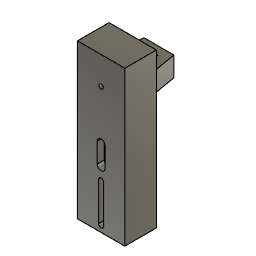
Seitenhalterung für vorne links v17 (Autodesk Fusion 360 design; units mm, degrees)
Autodesk Fusion 360 part; units mm, degrees
sketch "Skizze1" plane through (0, 0, 0) normal (0, 0, 1) x (1, 0, 0)
  line L0 (30, 20) -> (-30, 20)
  line L1 (-30, 20) -> (-30, -20)
  line L2 (-30, -20) -> (30, -20)
  line L3 (30, -20) -> (30, 20)
  line L4 (30, 20) -> (-30, -20) construction
  line L5 (-30, 20) -> (30, -20) construction
  dimension "d2" = 60
  dimension "d3" = 40
  constraint perpendicular L0 L1
  constraint parallel L0 L2
  constraint parallel L1 L3
  constraint horizontal L0
  constraint coincident L4 origin
  constraint coincident L5 origin
  measures "d2" distance of L1.end L2.end
  measures "d3" distance of L0.end L1.end
extrude "Extrusion1" add sketch "Skizze1" along normal blind 195 makes body 1
sketch "Skizze3" plane through (0, -20, 0) normal (0, -1, 0) x (1, 0, 0)
  line L0 (-30, 0) -> (30, 0)
  line L1 (30, 0) -> (30, 195)
  line L2 (30, 195) -> (-30, 195)
  line L3 (-30, 195) -> (-30, 0)
  line L4 (3.1, 8.1) -> (3.1, 56.9)
  arc A0 (3.1, 56.9) -> (-3.1, 56.9) centre (0, 56.9) ccw
  line L5 (-3.1, 56.9) -> (-3.1, 8.1)
  arc A1 (-3.1, 8.1) -> (3.1, 8.1) centre (0, 8.1) ccw
  line L6 (0, 5) -> (0, 60) construction
  line L7 (2.5, 72.5) -> (2.5, 97.5)
  arc A2 (2.5, 97.5) -> (-2.5, 97.5) centre (0, 97.5) ccw
  line L8 (-2.5, 97.5) -> (-2.5, 72.5)
  arc A3 (-2.5, 72.5) -> (2.5, 72.5) centre (0, 72.5) ccw
  line L9 (0, 70) -> (0, 100) construction
  point P0 (0, 195)
  dimension "d52" = 6.2
  dimension "d53" = 5
  constraint midpoint L2 P0
  constraint tangent L4 A0
  constraint tangent A0 L5
  constraint parallel L4 L5
  constraint tangent L5 A1
  constraint tangent L4 A1
  constraint midpoint A1 L6.start
  constraint midpoint A0 L6.end
  constraint vertical L6
  constraint tangent L7 A2
  constraint tangent A2 L8
  constraint parallel L7 L8
  constraint tangent L8 A3
  constraint tangent L7 A3
  constraint midpoint A3 L9.start
  constraint midpoint A2 L9.end
  constraint parallel L3 L9
  measures "d52" diameter of A0
  measures "d53" diameter of A2
extrude "Extrusion2" cut sketch "Skizze3" against normal blind 40 contours L4 A0 L5 A1 | L7 A2 L8 A3 bodies 1
sketch "Skizze4" plane through (30, 0, 0) normal (1, 0, 0) x (0, 1, 0)
  line L0 (-20, 0) -> (20, 0)
  line L1 (20, 0) -> (20, 195)
  line L2 (20, 195) -> (-20, 195)
  line L3 (-20, 195) -> (-20, 0)
  circle A0 centre (0, 174.5) radius 4.15
  dimension "d12" = 8.3
  measures "d12" diameter of A0
extrude "Extrusion3" add sketch "Skizze4" against normal blind 60 separate body contours A0 makes body 2
sketch "Skizze6" plane through (0, 0, 0) normal (0, 1, 0) x (1, 0, 0)
sketch "Skizze7" plane through (0, 20, 0) normal (0, 1, 0) x (-1, 0, 0)
  line L0 (-30, 0) -> (30, 0)
  line L1 (30, 0) -> (30, 195)
  line L2 (30, 195) -> (-30, 195)
  line L3 (-30, 195) -> (-30, 0)
  circle A0 centre (0, 160) radius 2.75
  line L4 (-2.5, 72.5) -> (-2.5, 97.5)
  arc A1 (2.5, 97.5) -> (-2.5, 97.5) centre (0, 97.5) ccw
  line L5 (2.5, 97.5) -> (2.5, 72.5)
  arc A2 (-2.5, 72.5) -> (2.5, 72.5) centre (0, 72.5) ccw
  line L6 (-3.1, 8.1) -> (-3.1, 56.9)
  arc A3 (3.1, 56.9) -> (-3.1, 56.9) centre (0, 56.9) ccw
  line L7 (3.1, 56.9) -> (3.1, 8.1)
  arc A4 (-3.1, 8.1) -> (3.1, 8.1) centre (0, 8.1) ccw
  dimension "d17" = 5.5
  measures "d17" diameter of A0
extrude "Extrusion4" cut sketch "Skizze7" against normal blind 40 contours A0 bodies 1
sketch "Skizze8" plane through (0, 20, 0) normal (0, 1, 0) x (-1, 0, 0)
  circle A0 centre (0, 160) radius 2.75
  line L0 (-30, 0) -> (30, 0)
  line L1 (30, 0) -> (30, 195)
  line L2 (30, 195) -> (-30, 195)
  line L3 (-30, 195) -> (-30, 0)
  circle A1 centre (0, 160) radius 6.65
  line L4 (-2.5, 72.5) -> (-2.5, 97.5)
  arc A2 (2.5, 97.5) -> (-2.5, 97.5) centre (0, 97.5) ccw
  line L5 (2.5, 97.5) -> (2.5, 72.5)
  arc A3 (-2.5, 72.5) -> (2.5, 72.5) centre (0, 72.5) ccw
  line L6 (-3.1, 8.1) -> (-3.1, 56.9)
  arc A4 (3.1, 56.9) -> (-3.1, 56.9) centre (0, 56.9) ccw
  line L7 (3.1, 56.9) -> (3.1, 8.1)
  arc A5 (-3.1, 8.1) -> (3.1, 8.1) centre (0, 8.1) ccw
  dimension "d20" = 13.3
  constraint concentric A0 A1
  measures "d20" diameter of A1
extrude "Extrusion5" cut sketch "Skizze8" against normal blind 4 contours A1 bodies 1
sketch "Skizze10" plane through (0, 20, 0) normal (0, 1, 0) x (-1, 0, 0)
  circle A0 centre (0, 160) radius 6.65
  line L0 (-30, 0) -> (30, 0)
  line L1 (30, 0) -> (30, 195)
  line L2 (30, 195) -> (-30, 195)
  line L3 (-30, 195) -> (-30, 0)
  line L4 (-14, 172.5) -> (-21, 172.5)
  line L5 (-21, 172.5) -> (-21, 147.5)
  line L6 (-21, 147.5) -> (-14, 147.5)
  line L7 (-14, 147.5) -> (-14, 172.5)
  line L8 (-2.5, 72.5) -> (-2.5, 97.5)
  arc A1 (2.5, 97.5) -> (-2.5, 97.5) centre (0, 97.5) ccw
  line L9 (2.5, 97.5) -> (2.5, 72.5)
  arc A2 (-2.5, 72.5) -> (2.5, 72.5) centre (0, 72.5) ccw
  line L10 (-3.1, 8.1) -> (-3.1, 56.9)
  arc A3 (3.1, 56.9) -> (-3.1, 56.9) centre (0, 56.9) ccw
  line L11 (3.1, 56.9) -> (3.1, 8.1)
  arc A4 (-3.1, 8.1) -> (3.1, 8.1) centre (0, 8.1) ccw
  dimension "d27" = 7
  dimension "d28" = 25
  constraint horizontal L4
  constraint vertical L5
  constraint horizontal L6
  constraint vertical L7
  measures "d27" distance of L4.start L4.end
  measures "d28" distance of L4.start L6.end
extrude "Extrusion7" add sketch "Skizze10" along normal blind 25 contours L4 L5 L6 L7 bodies 1
sketch "Skizze11" plane through (14, 0, 0) normal (-1, 0, 0) x (0, -1, 0)
  line L0 (-20, 147.5) -> (-20, 172.5)
  line L1 (-20, 172.5) -> (-45, 172.5)
  line L2 (-45, 172.5) -> (-45, 147.5)
  line L3 (-45, 147.5) -> (-20, 147.5)
  line L4 (-45, 172.5) -> (-38, 172.5)
  line L5 (-38, 172.5) -> (-38, 147.5)
  line L6 (-38, 147.5) -> (-45, 147.5)
  line L7 (-45, 147.5) -> (-45, 172.5)
  dimension "d31" = 7
  dimension "d32" = 25
  constraint horizontal L4
  constraint vertical L5
  constraint horizontal L6
  constraint vertical L7
  constraint coincident L1.end L2.start
  measures "d31" distance of L1.end L4.end
  measures "d32" distance of L1.end L2.end
sketch "Skizze12" plane through (0, 20, 0) normal (0, 1, 0) x (-1, 0, 0)
  line L0 (-14, 147.5) -> (-21, 147.5)
  line L1 (-21, 147.5) -> (-21, 172.5)
  line L2 (-21, 172.5) -> (-14, 172.5)
  line L3 (-14, 172.5) -> (-14, 147.5)
  circle A0 centre (0, 160) radius 6.65
  line L4 (-30, 0) -> (30, 0)
  line L5 (30, 0) -> (30, 195)
  line L6 (30, 195) -> (-30, 195)
  line L7 (-30, 195) -> (-30, 0)
  line L8 (0, 141) -> (23.4993, 141)
  arc A1 (23.4993, 141) -> (23.4993, 144) centre (23.4993, 142.5) ccw
  line L9 (23.4993, 144) -> (0, 144)
  arc A2 (0, 144) -> (0, 141) centre (0, 142.5) ccw
  line L10 (0, 142.5) -> (23.4993, 142.5) construction
  line L11 (0.0369, 132) -> (23.5, 132)
  arc A3 (23.5, 132) -> (23.5, 135) centre (23.5, 133.5) ccw
  line L12 (23.5, 135) -> (0.0369, 135)
  arc A4 (0.0369, 135) -> (0.0369, 132) centre (0.0369, 133.5) ccw
  line L13 (0.0369, 133.5) -> (23.5, 133.5) construction
  line L14 (-2.5, 72.5) -> (-2.5, 97.5)
  arc A5 (2.5, 97.5) -> (-2.5, 97.5) centre (0, 97.5) ccw
  line L15 (2.5, 97.5) -> (2.5, 72.5)
  arc A6 (-2.5, 72.5) -> (2.5, 72.5) centre (0, 72.5) ccw
  line L16 (-3.1, 8.1) -> (-3.1, 56.9)
  arc A7 (3.1, 56.9) -> (-3.1, 56.9) centre (0, 56.9) ccw
  line L17 (3.1, 56.9) -> (3.1, 8.1)
  arc A8 (-3.1, 8.1) -> (3.1, 8.1) centre (0, 8.1) ccw
  point P0 (0, 142.5)
  point P1 (27.5, 142.75)
  dimension "d38" = 3
  dimension "d39" = 3
  constraint tangent L8 A1
  constraint tangent A1 L9
  constraint parallel L8 L9
  constraint tangent L9 A2
  constraint tangent L8 A2
  constraint horizontal L10
  constraint tangent L11 A3
  constraint tangent A3 L12
  constraint parallel L11 L12
  constraint tangent L12 A4
  constraint tangent L11 A4
  constraint perpendicular L5 L13
  constraint coincident P0 A2.centre
  measures "d38" diameter of A1
  measures "d39" diameter of A3
extrude "Extrusion8" add sketch "Skizze11" along normal blind 28 contours L1 L2 L3 L4 L5 L6 L7 bodies 1
sketch "Skizze13" plane through (0, 45, 0) normal (0, 1, 0) x (-1, 0, 0)
  line L0 (14, 172.5) -> (-21, 172.5)
  line L1 (-21, 172.5) -> (-21, 147.5)
  line L2 (-21, 147.5) -> (14, 147.5)
  line L3 (14, 147.5) -> (14, 172.5)
  circle A0 centre (0, 160) radius 2.75
  dimension "d35" = 5.5
  measures "d35" diameter of A0
extrude "Extrusion9" cut sketch "Skizze13" against normal blind 10 contours A0 bodies 1
extrude "Extrusion10" cut sketch "Skizze12" against normal blind 1 contours L8 A1 L9 A2 | L11 A3 L12 A4 bodies 1
extrude "Extrusion11" add 1 faces at (21, 28.3333, 164.1667) along direction (1, 0, 0) blind 3 on bodies 1 bodies 1
extrude "Extrusion12" add 1 faces at (16.9167, 45, 160) along direction (0, 1, 0) blind 3 on bodies 1 bodies 1
draft "Entwurf1" angle 10 neutral plane through (21, 48, 172.5) pull (0, 1, 0) 1 faces at (24, 38.6667, 164.1667) on bodies 1
draft "Entwurf2" angle 10 neutral plane through (14, 38, 172.5) pull (0, -1, 0) 1 faces at (14, 26, 155.8333) on bodies 1
sketch "Skizze14" plane through (0, -20, 0) normal (0, -1, 0) x (1, 0, 0)
  circle A0 centre (0, 160) radius 2.75
  line L0 (-30, 0) -> (30, 0)
  line L1 (30, 0) -> (30, 195)
  line L2 (30, 195) -> (-30, 195)
  line L3 (-30, 195) -> (-30, 0)
  line L4 (2.5, 97.5) -> (2.5, 72.5)
  arc A1 (-2.5, 72.5) -> (2.5, 72.5) centre (0, 72.5) ccw
  line L5 (-2.5, 72.5) -> (-2.5, 97.5)
  arc A2 (2.5, 97.5) -> (-2.5, 97.5) centre (0, 97.5) ccw
  line L6 (3.1, 56.9) -> (3.1, 8.1)
  arc A3 (-3.1, 8.1) -> (3.1, 8.1) centre (0, 8.1) ccw
  line L7 (-3.1, 8.1) -> (-3.1, 56.9)
  arc A4 (3.1, 56.9) -> (-3.1, 56.9) centre (0, 56.9) ccw
  line L8 (-5, 97.5) -> (-5, 72.5)
  arc A5 (-5, 72.5) -> (5, 72.5) centre (0, 72.5) ccw
  line L9 (5, 72.5) -> (5, 97.5)
  arc A6 (5, 97.5) -> (-5, 97.5) centre (0, 97.5) ccw
  line L10 (0, 97.5) -> (0, 72.5) construction
  dimension "d54" = 10
  constraint tangent L8 A5
  constraint tangent A5 L9
  constraint parallel L8 L9
  constraint tangent L9 A6
  constraint tangent L8 A6
  constraint coincident A1.centre A5.centre
  constraint vertical L10
  constraint coincident A2.centre A6.centre
  measures "d54" diameter of A5
extrude "Extrusion13" cut sketch "Skizze14" against normal blind 9 contours L8 A5 L9 A6 bodies 1
extrude "Extrusion14" cut 1 faces at (-30, -1.0141, 173.1467) along direction (1, 0, 0) blind 50 on bodies 2 bodies 1 2
combine "Kombinieren1" operation add target body 1 tool bodies 2
sketch "Skizze15" plane through (0, 38, 0) normal (0, -1, 0) x (1, 0, 0)
  circle A0 centre (0, 160) radius 2.75
  line L0 (14, 147.5) -> (14, 172.5)
  line L1 (14, 172.5) -> (-14, 172.5)
  line L2 (-14, 172.5) -> (-14, 147.5)
  line L3 (-14, 147.5) -> (14, 147.5)
  circle A1 centre (0, 160) radius 6.65
  dimension "d59" = 13.3
  constraint concentric A0 A1
  measures "d59" diameter of A1
extrude "Extrusion15" cut sketch "Skizze15" against normal blind 4 contours A1 bodies 1
